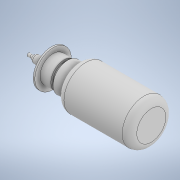
# Autodesk Inventor part: Part6
Saved by Autodesk Inventor 2021 (Build 250183000, 183)
## iProperties
Created: 2021-01-27
Part Number: Part6
Material: Generic
Document SubType Name: Modeling
Designer: Emil
Density: 1 g/cm^3
Appearance: Default
Author: Emil
Autodesk Inventor part; units mm, degrees
ref_plane "YZ Plane" through (0, 0, 0) normal (1, 0, 0) x (0, 1, 0)
ref_plane "XZ Plane" through (0, 0, 0) normal (0, 1, 0) x (-1, 0, 0)
ref_plane "XY Plane" through (0, 0, 0) normal (0, 0, 1) x (1, 0, 0)
sketch "Sketch2" plane through (0, 0, 0) normal (0, 1, 0) x (-1, 0, 0)
  line L0 (-1, 3) -> (-9, 3)
  line L1 (-10, 2) -> (-10, -2)
  line L2 (-9, -3) -> (-1, -3)
  line L3 (0, 0) -> (0, 2)
  arc A0 (-10, -2) -> (-9, -3) centre (-9, -2) ccw
  arc A1 (-9, 3) -> (-10, 2) centre (-9, 2) ccw
  arc A2 (-1, -3) -> (0, -2) centre (-1, -2) ccw
  arc A3 (0, 2) -> (-1, 3) centre (-1, 2) ccw
  line L4 (0, 2) -> (1.5, 2)
  line L5 (1.5, -2) -> (0, -2)
  line L6 (0, 0) -> (0, 2)
  line L7 (1.5, 1.4302) -> (2, 1.4302)
  line L8 (2, 1.4302) -> (2, 0)
  line L9 (2, -1.5) -> (1.5, -1.5)
  line L10 (1.5, 0) -> (1.5, 1.4302)
  line L11 (3.5, 1.8) -> (2, 1.8)
  line L12 (2, -1.8) -> (3.5, -1.8)
  line L13 (3.5, 0) -> (3.5, 1.8)
  line L14 (3.7281, 2.5) -> (3.5, 2.5)
  line L15 (3.5, -2.5) -> (3.7281, -2.5)
  line L16 (4.7281, 0.65) -> (3.7281, 0.65)
  line L17 (3.7281, 0.65) -> (3.7281, 0)
  line L18 (3.7281, -0.65) -> (4.6944, -0.65)
  line L19 (4.7614, -0.6455) -> (5.8082, -0.5038)
  line L20 (6.0942, -0.3624) -> (6.0942, -0.3624)
  line L21 (6.4473, -0.2165) -> (6.8473, -0.2165)
  line L22 (6.8473, -0.2165) -> (6.8473, 0)
  arc A4 (6.4473, -0.2165) -> (6.0942, -0.3624) centre (6.4473, -0.7165) ccw
  arc A5 (5.8082, -0.5038) -> (6.0942, -0.3624) centre (5.7412, -0.0084) ccw
  arc A6 (4.6944, -0.65) -> (4.7614, -0.6455) centre (4.6944, -0.15) ccw
  line L23 (6.8473, 0) -> (-10, 0)
  line L24 (1.5, 2) -> (1.5, 0)
  line L25 (1.5, -1.5) -> (1.5, -2)
  line L26 (2, 1.8) -> (2, 0)
  line L27 (2, -1.5) -> (2, -1.8)
  line L28 (3.5, 2.5) -> (3.5, 0)
  line L29 (3.5, -1.8) -> (3.5, -2.5)
  line L30 (3.7281, -2.5) -> (3.7281, -0.65)
  line L31 (3.7281, 0.65) -> (3.7281, 2.5)
  line L32 (4.7281, -0.65) -> (4.7281, -0.6489)
  line L33 (4.7281, 0) -> (4.7281, 0.65)
  point P0 (0, 0)
  point P1 (0, 3)
  point P2 (-10, -3)
  point P3 (0, -3)
  point P4 (0, -2)
  dimension "d0" = 3
  dimension "d1" = 6
  dimension "d2" = 10
  dimension "d3" = 1
  dimension "d4" = 1.5
  dimension "d5" = 4
  dimension "d6" = 3.6
  dimension "d7" = 1.5
  dimension "d8" = 0.5
  dimension "d9" = 1.8
  dimension "d10" = 1.5
  dimension "d11" = 5
  dimension "d12" = 2.5
  dimension "d13" = 1
  dimension "d14" = 1.3
  dimension "d15" = 0.65
  dimension "d16" = 0.5
  dimension "d18" = 0.4
  dimension "d56" = 3.3473
  dimension "d59" = 1.6467
  dimension "d63" = 6.8473
  dimension "d64" = 1.7835
  constraints: 68 end point, 19 parallel, 17 point on line, 15 point on circle, 15 tangent, 10 perpendicular, 7 centre point, 7 horizontal, 5 equal radius, 1 midpoint
  measures "d0" distance from line of point (0, 0) L0
  measures "d1" distance of point (0, -3) point (0, 3)
  measures "d2" distance of point (-10, -3) point (0, -3)
  measures "d3" radius of A0
  measures "d4" distance of L3.end L4.end
  measures "d5" distance of L5.end L3.end
  measures "d6" distance of L12.end L11.start
  measures "d7" distance of L12.start L12.end
  measures "d8" distance of L9.start L9.end
  measures "d9" distance from line of L12 point (0, 0)
  measures "d10" distance from line of point (0, 0) L9
  measures "d11" distance of L15.end L14.start
  measures "d12" vertical distance of point (0, 0) L14.start
  measures "d13" distance of L18.start L32.start
  measures "d14" distance of L32.start L16.start
  measures "d15" distance from line of point (0, 0) L18
  measures "d16" radius of A4
  measures "d18" distance of L21.start L21.end
  measures "d56" distance between parallel lines of L22 L13
  measures "d59" distance between parallel lines of L21 L7
  measures "d63" distance from line of point (0, -2) L22
  measures "d64" distance from line of point (0, -2) L21
revolve "Revolution1" add sketch "Sketch2" angle 360 about axis through (-6.8473, 0, 0) along (1, 0, 0) contours L23 L22 L21 A4 A5 L19 A6 L18 L30 L15 L29 L12 L27 L9 L25 L5 A2 L2 A0 L1
body "Solid1"
